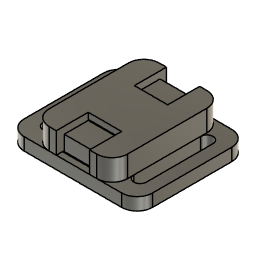
SquidSlimeCaseAUX (Autodesk Fusion 360 design; units mm, degrees)
Autodesk Fusion 360 part; units mm, degrees
sketch "スケッチ1" plane through (0, 0, 0) normal (0, 0, 1) x (1, 0, 0)
  line L0 (52.54, 69.52) -> (67.78, 69.52)
  line L1 (70.32, 72.06) -> (70.32, 97.46)
  line L2 (67.78, 100) -> (52.54, 100)
  line L3 (50, 97.46) -> (50, 72.06)
  arc A0 (52.54, 100) -> (50, 97.46) centre (52.54, 97.46) ccw
  arc A1 (70.32, 97.46) -> (67.78, 100) centre (67.78, 97.46) ccw
  arc A2 (67.78, 69.52) -> (70.32, 72.06) centre (67.78, 72.06) ccw
  arc A3 (50, 72.06) -> (52.54, 69.52) centre (52.54, 72.06) ccw
  circle A4 centre (52.54, 97.46) radius 1
  circle A5 centre (67.78, 97.46) radius 1
  circle A6 centre (67.78, 72.06) radius 1
  circle A7 centre (52.54, 72.06) radius 1
  line L4 (60.16, 92.4) -> (60.16, 77.12)
  line L5 (65.24, 92.4) -> (55.08, 92.4)
  line L6 (55.08, 77.12) -> (65.24, 77.12)
  line L7 (55.08, 100) -> (55.08, 92.4)
  line L8 (55.08, 77.12) -> (55.08, 69.52)
  line L9 (65.24, 100) -> (65.24, 92.4)
  line L10 (65.24, 77.12) -> (65.24, 69.52)
  dimension "d7" = 2.54
  dimension "d8" = 2
  dimension "d9" = 2
  dimension "d10" = 2
  dimension "d11" = 2
  constraint horizontal L0
  constraint vertical L1
  constraint horizontal L2
  constraint vertical L3
  constraint tangent L2 A0
  constraint tangent L3 A0
  constraint tangent L1 A1
  constraint tangent L2 A1
  constraint equal A0 A1
  constraint tangent L0 A2
  constraint tangent L1 A2
  constraint equal A0 A2
  constraint tangent L3 A3
  constraint tangent L0 A3
  constraint equal A0 A3
  constraint concentric A0 A4
  constraint concentric A1 A5
  constraint concentric A2 A6
  constraint concentric A3 A7
  constraint coincident L6.start L7
  constraint collinear L7 L8
  constraint coincident L6 L4.end
  constraint coincident L6.end L9
  constraint collinear L9 L10
  constraint coincident L5 L4.start
  measures "d7" radius of A0
  measures "d8" diameter of A4
  measures "d9" diameter of A5
  measures "d10" diameter of A6
  measures "d11" diameter of A7
extrude "押し出し1" add sketch "スケッチ1" along normal blind 4.8 contours L0 L6 L8 L10 | L2 L5 L7 L9 makes body 1 at (61.8533, 94.9333, 0) makes body 2 at (58.4667, 72.0533, 0)
extrude "押し出し2" add 1 faces at (58.4667, 69.52, 3.2) along direction (0, -1, 0) blind 0.1 on bodies 2 bodies 2
extrude "押し出し3" add 1 faces at (61.8533, 100, 3.2) along direction (0, 1, 0) blind 0.1 on bodies 1 bodies 1
extrude "押し出し4" add sketch "スケッチ1" against normal blind 1 separate body makes body 3
combine "結合1" operation add target body 3 tool bodies 1 2
sketch "スケッチ2" plane through (0, 0, -1) normal (0, 0, -1) x (1, 0, 0)
  circle A0 centre (67.78, -72.06) radius 1
  circle A1 centre (52.54, -72.06) radius 1
  circle A2 centre (67.78, -97.46) radius 1
  circle A3 centre (52.54, -97.46) radius 1
  arc A4 (52.54, -69.52) -> (50, -72.06) centre (52.54, -72.06) ccw
  line L0 (50, -72.06) -> (50, -97.46)
  arc A5 (50, -97.46) -> (52.54, -100) centre (52.54, -97.46) ccw
  line L1 (52.54, -100) -> (67.78, -100)
  arc A6 (67.78, -100) -> (70.32, -97.46) centre (67.78, -97.46) ccw
  line L2 (70.32, -97.46) -> (70.32, -72.06)
  arc A7 (70.32, -72.06) -> (67.78, -69.52) centre (67.78, -72.06) ccw
  line L3 (67.78, -69.52) -> (52.54, -69.52)
  line L4 (52.54, -100.4) -> (67.78, -100.4)
  arc A8 (67.78, -100.4) -> (70.72, -97.46) centre (67.78, -97.46) ccw
  line L5 (70.72, -97.46) -> (70.72, -72.06)
  arc A9 (70.72, -72.06) -> (67.78, -69.12) centre (67.78, -72.06) ccw
  line L6 (67.78, -69.12) -> (52.54, -69.12)
  arc A10 (52.54, -69.12) -> (49.6, -72.06) centre (52.54, -72.06) ccw
  line L7 (49.6, -72.06) -> (49.6, -97.46)
  arc A11 (49.6, -97.46) -> (52.54, -100.4) centre (52.54, -97.46) ccw
  line L8 (52.54, -102.4) -> (67.78, -102.4)
  arc A12 (67.78, -102.4) -> (72.72, -97.46) centre (67.78, -97.46) ccw
  line L9 (72.72, -97.46) -> (72.72, -72.06)
  arc A13 (72.72, -72.06) -> (67.78, -67.12) centre (67.78, -72.06) ccw
  line L10 (67.78, -67.12) -> (52.54, -67.12)
  arc A14 (52.54, -67.12) -> (47.6, -72.06) centre (52.54, -72.06) ccw
  line L11 (47.6, -72.06) -> (47.6, -97.46)
  arc A15 (47.6, -97.46) -> (52.54, -102.4) centre (52.54, -97.46) ccw
  line L12 (60.16, -67.12) -> (60.16, -102.4)
  line L13 (55.08, -67.12) -> (55.08, -102.4)
  line L14 (65.24, -67.12) -> (65.24, -102.4)
  dimension "d24" = 0.4
  dimension "d25" = 2.4
  dimension "d58" = 5.08
  dimension "d59" = -5.08
  constraint midpoint L10 L12.start
  constraint midpoint L8 L12.end
extrude "押し出し5" add sketch "スケッチ2" against normal blind 1 separate body contours L6 L10 L12 L13 | L4 L6 A10 L7 A11 L8 L10 A14 L11 A15 L13 | L6 L10 L12 L14 | L4 L8 L12 L13 | L4 A8 L5 A9 L6 L8 A12 L9 A13 L10 L14 | L4 L8 L12 L14 makes body 4
extrude "押し出し6" add sketch "スケッチ2" along normal blind 1 bodies 4
extrude "押し出し7" add sketch "スケッチ2" along normal blind 1 contours A0 | A1 | A2 | A3 bodies 4
extrude "押し出し8" add sketch "スケッチ2" against normal blind 8 separate body contours A0 | A1 | A2 | A3 | A4 L0 A5 L1 L3 L13 | A4 L0 A5 L1 L3 L4 L6 A10 L7 A11 L13 | L3 L6 L12 L13 | L1 L3 L12 L13 | L3 L6 L12 L14 | L1 L3 L12 L14 | L6 L10 L12 L13 | L4 L6 A10 L7 A11 L8 L10 A14 L11 A15 L13 | L1 L4 L12 L13 | L1 A6 L2 A7 L3 L4 A8 L5 A9 L6 L14 | L1 A6 L2 A7 L3 L14 | L6 L10 L12 L14 | L1 L4 L12 L14 | L4 L8 L12 L13 | L4 A8 L5 A9 L6 L8 A12 L9 A13 L10 L14 | L4 L8 L12 L14 makes body 5
extrude "押し出し9" cut 1 faces at (64.3467, 88.9933, -1) along direction (0, 0, 1) blind 1 on bodies 5 bodies 5
extrude "押し出し10" cut 2 faces at (61.8533, 94.9667, 4.8) (58.4667, 71.9867, 4.8) along direction (0, 0, 1) blind 7 on bodies 3 bodies 5
extrude "押し出し11" cut 1 faces at (58.4667, 69.42, 5.5333) along direction (0, -1, 0) blind 10 on bodies 5 bodies 5
extrude "押し出し12" cut 1 faces at (61.8533, 100.1, 5.5333) along direction (0, 1, 0) blind 11 on bodies 5 bodies 5
extrude "押し出し13" cut 1 faces at (61.8533, 100.1, 3.2) along direction (0, 1, 0) blind 8 on bodies 3 bodies 5
extrude "押し出し14" cut 1 faces at (58.4667, 69.42, 3.2) along direction (0, -1, 0) blind 9 on bodies 3 bodies 5
extrude "押し出し15" cut sketch "スケッチ2" against normal blind 5.8 contours A0 | A1 | A2 | A3 | A4 L0 A5 L1 L3 L13 | A4 L0 A5 L1 L3 L4 L6 A10 L7 A11 L13 | L3 L6 L12 L13 | L1 L3 L12 L13 | L3 L6 L12 L14 | L1 L3 L12 L14 | L1 L4 L12 L13 | L1 A6 L2 A7 L3 L4 A8 L5 A9 L6 L14 | L1 A6 L2 A7 L3 L14 | L1 L4 L12 L14 bodies 5
extrude "押し出し16" cut 2 faces at (65.24, 98.4, 6.2667) (65.24, 71.12, 6.2667) along direction (1, 0, 0) blind 0.25 on bodies 5 bodies 5
extrude "押し出し17" cut 2 faces at (55.08, 71.12, 6.2667) (55.08, 98.4, 6.2667) along direction (-1, 0, 0) blind 0.25 on bodies 5 bodies 5
extrude "押し出し18" cut 1 faces at (61.9367, 92.4, 6.2667) along direction (0, -1, 0) blind 0.25 on bodies 5 bodies 5
extrude "押し出し19" cut 1 faces at (61.9367, 77.12, 5.5333) along direction (0, 1, 0) blind 0.25 on bodies 5 bodies 5
extrude "押し出し20" cut sketch "スケッチ1" against normal blind 12 contours A4 | A5 | A6 | A7 bodies 4
extrude "押し出し21" add sketch "スケッチ2" against normal blind 5.8 contours A4 L0 A5 L1 L3 L13 | A4 L0 A5 L1 L3 L4 L6 A10 L7 A11 L13 | L1 A6 L2 A7 L3 L4 A8 L5 A9 L6 L14 | L1 A6 L2 A7 L3 L14 bodies 5
extrude "押し出し22" cut 2 faces at (69.8618, 88.683, -1) (50.4582, 88.683, -1) along direction (0, 0, 1) blind 1 on bodies 5 bodies 5
extrude "押し出し23" cut 1 faces at (65.24, 82.2967, 1.6) along direction (1, 0, 0) blind 0.25 on bodies 5 bodies 5
extrude "押し出し24" cut 1 faces at (55.08, 82.2967, 1.6) along direction (-1, 0, 0) blind 0.25 on bodies 5 bodies 5
extrude "押し出し25" cut 1 faces at (58.3833, 87.2233, 7) along direction (0, 0, -1) blind 0.2 on bodies 5 bodies 5
extrude "押し出し26" add 1 faces at (57.7867, 88.7047, -2) along direction (0, 0, -1) blind 1.5 separate body on bodies 4 makes body 6
move_face "面をオフセット1" offset -0.75 4 faces at (51.8783, 71.3102, -3) (53.5091, 97.7068, -3) (67.014, 96.8172, -3) (68.7491, 72.3068, -3) on bodies 6
combine "結合2" operation add target body 4 tool bodies 6
extrude "押し出し27" add 1 faces at (57.9117, 88.4882, -3.5) along direction (0, 0, -1) blind 0.5 on bodies 4 bodies 4
sketch "スケッチ3" plane through (0, 0, -4) normal (0, 0, -1) x (1, 0, 0)
  circle A0 centre (52.54, -97.46) radius 1.75
  circle A1 centre (52.54, -72.06) radius 1.75
  circle A2 centre (67.78, -97.46) radius 1.75
  circle A3 centre (67.78, -72.06) radius 1.75
  arc A4 (47.6, -97.46) -> (52.54, -102.4) centre (52.54, -97.46) ccw
  line L0 (52.54, -102.4) -> (67.78, -102.4)
  arc A5 (67.78, -102.4) -> (72.72, -97.46) centre (67.78, -97.46) ccw
  line L1 (72.72, -97.46) -> (72.72, -72.06)
  arc A6 (72.72, -72.06) -> (67.78, -67.12) centre (67.78, -72.06) ccw
  line L2 (67.78, -67.12) -> (52.54, -67.12)
  arc A7 (52.54, -67.12) -> (47.6, -72.06) centre (52.54, -72.06) ccw
  line L3 (47.6, -72.06) -> (47.6, -97.46)
  line L4 (76.72, -97.46) -> (76.72, -74.06)
  line L5 (80.72, -97.46) -> (80.72, -72.06)
  line L6 (43.6, -74.06) -> (43.6, -97.46)
  line L7 (39.6, -72.06) -> (39.6, -97.46)
  line L8 (60.16, -67.12) -> (60.16, -102.4)
  arc A8 (80.72, -72.06) -> (75.78, -67.12) centre (75.78, -72.06) ccw
  arc A9 (44.54, -67.12) -> (39.6, -72.06) centre (44.54, -72.06) ccw
  line L9 (44.54, -67.12) -> (75.78, -67.12)
  line L10 (47.6, -84.76) -> (72.72, -84.76)
  line L11 (47.6, -74.06) -> (47.6, -97.46)
  line L12 (72.72, -74.06) -> (72.72, -97.46)
  arc A10 (45.6, -72.06) -> (43.6, -74.06) centre (45.6, -74.06) ccw
  arc A11 (47.6, -74.06) -> (45.6, -72.06) centre (45.6, -74.06) ccw
  arc A12 (74.72, -72.06) -> (72.72, -74.06) centre (74.72, -74.06) ccw
  arc A13 (76.72, -74.06) -> (74.72, -72.06) centre (74.72, -74.06) ccw
  arc A14 (75.78, -102.4) -> (80.72, -97.46) centre (75.78, -97.46) ccw
  arc A15 (74.72, -97.46) -> (76.72, -95.46) centre (74.72, -95.46) ccw
  arc A16 (72.72, -95.46) -> (74.72, -97.46) centre (74.72, -95.46) ccw
  line L13 (44.54, -102.4) -> (75.78, -102.4)
  arc A17 (39.6, -97.46) -> (44.54, -102.4) centre (44.54, -97.46) ccw
  arc A18 (43.6, -95.46) -> (45.6, -97.46) centre (45.6, -95.46) ccw
  arc A19 (45.6, -97.46) -> (47.6, -95.46) centre (45.6, -95.46) ccw
  dimension "d76" = 8
  dimension "d78" = 8
  dimension "d79" = 2
  constraint midpoint L2 L8.start
  constraint midpoint L0 L8.end
  constraint symmetric L8 L5.end L7.start
  constraint symmetric L8 A8.end A9.start
  constraint symmetric L8 A8 A9
  constraint tangent A8 L9
  constraint midpoint L3 L10.start
  constraint midpoint L1 L10.end
  constraint coincident A4.start L3.end
  constraint coincident A5.end L1.start
  constraint tangent L6 A10
  constraint tangent L11 A11
  constraint equal A10 A11
  constraint coincident A10.start A11.end
  constraint tangent L12 A12
  constraint equal A10 A12
  constraint tangent L4 A13
  constraint equal A10 A13
  constraint coincident A12.start A13.end
  constraint symmetric L5.end L10 L5.start
  constraint symmetric A8.end L10 A14.start
  constraint symmetric A8 L10 A14
  constraint symmetric L7.start L10 L7.end
  constraint symmetric A9.start L10 L13.start
  constraint symmetric A9 L10 A17
  constraint symmetric L10 L6.start A18.start
  constraint symmetric L10 A10.start A18.end
  constraint symmetric L10 A10 A18
  constraint symmetric L10 L11.start A19.end
  constraint symmetric L10 A11 A19
  constraint symmetric L10 A12.start A15.start
  constraint symmetric L10 L12.start A16.start
  constraint symmetric L10 A12 A16
  constraint symmetric L10 L4.end A15.end
  constraint symmetric L10 A13 A15
  measures "d79" radius of A10
extrude "押し出し28" add sketch "スケッチ3" against normal blind 4 separate body contours A4 A7 L3 L6 L7 A9 L9 L11 A10 A11 L13 A17 A18 A19 | A5 L1 A6 L4 L5 A8 L9 L12 A12 A13 A14 A15 A16 L13 makes body 7 at (40.9333, 81.1933, 0) makes body 8 at (79.3867, 88.3267, -4)
combine "結合3" operation add target body 4 tool bodies 7 8
equation "d58 = ( 10.16 / 2 ) * 1 mm"
named bodies: "Mock", "SquidSlimeCaseAUXBottom", "SquidSlimeCaseAUXUpper"
